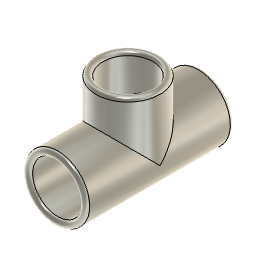
Pset2-PVCJoint (Autodesk Fusion 360 design; units mm, degrees)
Autodesk Fusion 360 part; units mm, degrees
note: some values were not read from the file. Set by a fixed rule: which face or edge a step refers to.
sketch "Sketch1" plane through (0, 0, 0) normal (0, 1, 0) x (1, 0, 0)
  circle A0 centre (0, 0) radius 10.75
  circle A1 centre (0, 0) radius 13.75
  dimension "d1" = 21.5
  dimension "d2" = 27.5
  constraint coincident A0.centre A1.centre
  constraint concentric A0 A1
  measures "d1" diameter of A0
  measures "d2" diameter of A1
extrude "Extrude1" add sketch "Sketch1" along normal blind 63.5
ref_plane "WorkPlane1" through (0, 18.5, 0) normal (0, 1, 0) x (0, 0, 1)
sketch "Sketch2" plane through (0, 18.5, 0) normal (0, 1, 0) x (1, 0, 0)
  circle A0 centre (0, 0) radius 10
  circle A1 centre (0, 0) radius 10.75
  dimension "d6" = 20
  dimension "d7" = 21.5
  constraint coincident A0.centre A1.centre
  constraint concentric A0 A1
  measures "d6" diameter of A0
  measures "d7" diameter of A1
extrude "Extrude2" add sketch "Sketch2" along normal blind 26.5
fillet "Fillet1" radius 1.5 1 edges at (-12.8195, 63.5, 4.9722)
fillet "Fillet2" radius 1.5 1 edges at (-10.0225, 63.5, -3.8874)
fillet "Fillet3" radius 1.5 1 edges at (-12.8195, 0, 4.9722)
fillet "Fillet4" radius 1.5 1 edges at (-10.0225, 0, -3.8874)
ref_plane "WorkPlane2" through (0, 0, 10) normal (0, 0, 1) x (1, 0, 0)
sketch "Sketch3" plane through (0, 0, 10) normal (0, 0, 1) x (1, 0, 0)
  line L0 (0, 0) -> (0, 31.75) construction
  circle A0 centre (0, 31.75) radius 10.75
  circle A1 centre (0, 31.75) radius 13.75
  dimension "d19" = 31.75
  dimension "d20" = 21.5
  dimension "d21" = 27.5
  constraint coincident L0.start origin
  constraint vertical L0
  constraint coincident L0.end A0.centre
  constraint concentric A0 A1
  measures "d19" distance of L0.start L0.end
  measures "d20" diameter of A0
  measures "d21" diameter of A1
extrude "Extrude3" add sketch "Sketch3" along normal blind 18
extrude "Extrude4" add 1 faces at (11.2787, 25.8512, 10) along direction (0, 0, -1) blind 10
extrude "Extrude5" add 1 faces at (-11.4002, 37.3943, 10) along direction (0, 0, -1) blind 10
sketch "Sketch4" plane through (0, 0, 0) normal (0, 0, 1) x (1, 0, 0)
  line L0 (0, 0) -> (0, 31.75) construction
  circle A0 centre (0, 31.75) radius 10
  dimension "d28" = 31.75
  dimension "d29" = 20
  constraint coincident L0.start origin
  constraint vertical L0
  constraint coincident L0.end A0.centre
  measures "d28" distance of L0.start L0.end
  measures "d29" diameter of A0
extrude "Extrude6" cut sketch "Sketch4" along normal blind 37
fillet "Fillet5" radius 1.5 1 edges at (-12.8195, 26.7778, 28)
fillet "Fillet6" radius 1.5 1 edges at (-10.0225, 35.6374, 28)
